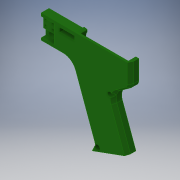
# Autodesk Inventor part: Griff_rechts
Saved by Autodesk Inventor 2019 (Build 230136000, 136)
## iProperties
Created: 2021-03-07
Part Number: Griff_rechts
Material: Generic
Document SubType Name: Modeling
Designer: Lukas
Density: 1 g/cm^3
Appearance: Default(3)
Author: Lukas
Autodesk Inventor part; units mm, degrees
ref_plane "YZ Plane" through (0, 0, 0) normal (1, 0, 0) x (0, 1, 0)
ref_plane "XZ Plane" through (0, 0, 0) normal (0, 1, 0) x (-1, 0, 0)
ref_plane "XY Plane" through (0, 0, 0) normal (0, 0, 1) x (1, 0, 0)
sketch "Sketch1" plane through (0, 0, 0) normal (0, 0, 1) x (1, 0, 0)
  line L0 (-51.5891, 42.2862) -> (-20.8072, -42.2862)
  line L1 (-20.8072, -42.2862) -> (-24.5184, -46.7089)
  line L2 (-24.5184, -46.7089) -> (-23.4923, -49.528)
  line L3 (-23.4923, -49.528) -> (23.4923, -32.427)
  line L4 (27.261, 47.2862) -> (1.261, 28.653)
  line L5 (1.261, 28.653) -> (23.4923, -32.427)
  line L6 (0, -74.8908) -> (0, 102.649) projected
  line L7 (-91.5891, 77.2862) -> (27.261, 77.2862)
  line L8 (27.261, 77.2862) -> (27.261, 47.2862)
  line L9 (-51.5891, 42.2862) -> (-91.5891, 42.2862)
  line L10 (-91.5891, 42.2862) -> (-91.5891, 77.2862)
  point P0 (0, 0)
  point P1 (-36.1981, 0)
  point P2 (0, -40.9775)
  dimension "d1" = 90
  dimension "d2" = 120
  dimension "d3" = 3
  dimension "d5" = 45
  dimension "d6" = 20
  dimension "d7" = 65
  dimension "d8" = 5
  dimension "d10" = 30
  dimension "d30" = 26
  dimension "d31" = 40
  dimension "d32" = 35
  constraints: 21 end point, 5 perpendicular, 2 midpoint, 1 horizontal, 1 horizontal alignment, 1 parallel, 1 vertical alignment
  measures "d1" distance of L0.start L0.end
  measures "d2" angle of L0 L1
  measures "d3" distance of L1.end L2.end
  measures "d5" distance between parallel lines of L5 L0
  measures "d6" angle of L6 L0
  measures "d7" distance of L4.end L3.end
  measures "d8" distance between parallel lines of L2 L0
  measures "d10" distance of L7.end L4.start
  measures "d30" distance from line of L8 L4.end
  measures "d31" distance of L0.start L9.end
  measures "d32" distance of L9.end L7.start
extrude "Extrusion1" add sketch "Sketch1" along normal blind 2.5
sketch "Sketch2" plane through (0, 0, 0) normal (0, 0, 1) x (1, 0, 0)
  line L0 (-51.5891, 42.2862) -> (-20.8072, -42.2862) projected
  line L1 (-20.8072, -42.2862) -> (-24.5184, -46.7089) projected
  line L2 (-24.5184, -46.7089) -> (-23.4923, -49.528) projected
  line L3 (-23.4923, -49.528) -> (23.4923, -32.427) projected
  line L4 (23.4923, -32.427) -> (1.261, 28.653) projected
  line L5 (1.261, 28.653) -> (27.261, 47.2862) projected
  line L6 (27.261, 47.2862) -> (27.261, 77.2862) projected
  line L7 (27.261, 77.2862) -> (-91.5891, 77.2862) projected
  circle A0 centre (-32, 28) radius 3
  circle A1 centre (-32, 28) radius 8.5
  line L8 (-91.5891, 77.2862) -> (-91.5891, 42.2862) projected
  line L9 (-91.5891, 42.2862) -> (-51.5891, 42.2862) projected
  point P0 (0, 0)
  dimension "d55" = 6
  dimension "d56" = 17
  dimension "d169" = 32
  dimension "d170" = 28
  constraints: 2 centre point, 1 coincident
  measures "d55" diameter of A0
  measures "d56" diameter of A1
  measures "d169" horizontal distance of A0.centre point (0, 0)
  measures "d170" vertical distance of point (0, 0) A0.centre
extrude "Extrusion2" add sketch "Sketch2" against normal blind 6 contours A1
sketch "Sketch3" plane through (0, 0, 0) normal (0, 0, 1) x (1, 0, 0)
  line L0 (-51.5891, 42.2862) -> (-20.8072, -42.2862) projected
  line L1 (-20.8072, -42.2862) -> (-24.5184, -46.7089) projected
  line L2 (-24.5184, -46.7089) -> (-23.4923, -49.528) projected
  line L3 (-23.4923, -49.528) -> (23.4923, -32.427) projected
  line L4 (23.4923, -32.427) -> (1.261, 28.653) projected
  line L5 (1.261, 28.653) -> (27.261, 47.2862) projected
  line L6 (27.261, 47.2862) -> (27.261, 77.2862) projected
  line L7 (27.261, 77.2862) -> (-91.5891, 77.2862) projected
  line L8 (-48.7882, 46.2862) -> (-16.4032, -42.6911)
  line L9 (-16.4032, -42.6911) -> (18.3655, -30.0363)
  line L10 (18.3655, -30.0363) -> (-3.5357, 30.1366)
  line L11 (-3.5357, 30.1366) -> (23.261, 49.3407)
  line L12 (23.261, 49.3407) -> (23.261, 77.2862)
  line L13 (27.261, 77.2862) -> (-91.5891, 77.2862) projected
  line L14 (1.261, 28.653) -> (27.261, 47.2862) projected
  line L15 (23.4923, -32.427) -> (1.261, 28.653) projected
  line L16 (-51.5891, 42.2862) -> (-20.8072, -42.2862) projected
  line L17 (-24.5184, -46.7089) -> (-20.8072, -42.2862) projected
  line L18 (-51.5891, 42.2862) -> (-20.8072, -42.2862)
  line L19 (-20.8072, -42.2862) -> (-24.5184, -46.7089)
  line L20 (-24.5184, -46.7089) -> (-23.4923, -49.528)
  line L21 (23.4923, -32.427) -> (-23.4923, -49.528)
  line L22 (-23.4923, -49.528) -> (23.4923, -32.427) projected
  line L23 (23.4923, -32.427) -> (1.261, 28.653)
  line L24 (1.261, 28.653) -> (27.261, 47.2862)
  line L25 (27.261, 77.2862) -> (27.261, 47.2862)
  line L26 (23.261, 77.2862) -> (27.261, 77.2862)
  line L27 (-91.5891, 77.2862) -> (-91.5891, 42.2862) projected
  line L28 (-91.5891, 42.2862) -> (-51.5891, 42.2862) projected
  line L29 (-91.5891, 77.2862) -> (-91.5891, 42.2862) projected
  line L30 (-51.5891, 42.2862) -> (-91.5891, 42.2862)
  line L31 (-91.5891, 42.2862) -> (-91.5891, 46.2862)
  line L32 (-91.5891, 46.2862) -> (-48.7882, 46.2862)
  point P0 (-51.5891, 77.2862)
  dimension "d20" = 4
  dimension "d21" = 4
  dimension "d22" = 4
  dimension "d23" = 4
  dimension "d24" = 4
  dimension "d33" = 4
  constraints: 32 end point, 6 perpendicular, 5 parallel, 2 point on line, 2 vertical, 1 collinear, 1 horizontal
  measures "d20" distance between parallel lines of L6 L12
  measures "d21" distance between parallel lines of L16 L8
  measures "d22" distance between parallel lines of L4 L10
  measures "d23" distance between parallel lines of L14 L11
  measures "d24" distance between parallel lines of L3 L9
  measures "d33" distance between parallel lines of L32 L28
extrude "Extrusion3" add sketch "Sketch3" against normal blind 10 contours L28 L27 L32 L8 L9 L10 L11 L12 L7 L6 L5 L4 L3 L2 L1 L0
fillet "Fillet7" radius 3 1 edges at (-40.5, 28, 0)
fillet "Fillet1" radius 6 2 edges at (7.4149, 0.0501, 0) (9.8627, 39.7386, 0)
fillet "Fillet3" radius 15 2 edges at (1.261, 28.653, -3.75) (-51.5891, 42.2862, -3.75)
fillet "Fillet2" radius 8 2 edges at (27.261, 47.2862, -3.75) (-20.8072, -42.2862, -3.75)
chamfer "Chamfer3" distance 3 angle 60 10 edges at (14.3227, -7.2338, 2.5) (4.9183, 27.5219, 2.5) (17.216, 40.0873, 2.5) (26.3772, 47.7401, 2.5) (27.261, 64.3407, 2.5) (-35.1919, -2.7647, 2.5) (-22.026, -42.0713, 2.5) (-24.1473, -46.2667, 2.5) (-53.4885, 39.5734, 2.5) (-76.8406, 42.2862, 2.5) measured on face at (-53.2017, 39.983, 2.5) measured on face at (26.761, 64.3407, 2.5) measured on face at (25.9325, 47.9685, 2.5) measured on face at (13.8529, -7.4048, 2.5) measured on face at (16.9247, 40.4937, 2.5) measured on face at (-76.8406, 42.7862, 2.5) measured on face at (4.4406, 27.6696, 2.5) measured on face at (-23.7642, -46.588, 2.5) measured on face at (-34.722, -2.5937, 2.5) measured on face at (-21.5336, -42.1581, 2.5)
sketch "Sketch4" plane through (0, 0, 0) normal (0, 0, 1) x (1, 0, 0)
  line L0 (-91.5891, 77.2862) -> (-91.5891, 46.2862) projected
  line L1 (-91.5891, 77.2862) -> (-42.0891, 77.2862)
  line L2 (-42.0891, 77.2862) -> (-42.0891, 60.2862)
  line L3 (-42.0891, 60.2862) -> (-91.5891, 60.2862)
  line L4 (-91.5891, 60.2862) -> (-91.5891, 77.2862)
  line L5 (24.261, 77.2862) -> (-91.5891, 77.2862) projected
  line L6 (-91.5891, 46.2862) -> (-48.7882, 46.2862) projected
  point P0 (0, 0)
  point P1 (11.261, 77.2862)
  point P2 (-76.5891, 52.2862)
  point P3 (-59.2913, 46.2862)
  point P4 (17.261, 77.2862)
  point P5 (27.261, 77.2862)
  dimension "d34" = 49.5
  dimension "d35" = 0
  dimension "d42" = 14
  constraints: 8 end point, 2 parallel, 1 horizontal, 1 perpendicular, 2 other
  measures "d34" distance of L1.start L1.end
  measures "d35" distance between parallel lines of L5 L1
  measures "d42" distance between parallel lines of L6 L3
extrude "Extrusion4" add sketch "Sketch4" against normal blind 10
chamfer "Chamfer1" distance 1 distance2 4 1 edges at (-42.0891, 77.2862, -5) measured on face at (-42.0891, 76.7862, -5)
chamfer "Chamfer4" distance 10 angle 45 1 edges at (-16.4032, -42.6911, -5)
sketch "Sketch5" plane through (-91.5891, 77.2862, 0) normal (-1, 0, 0) x (0, 0, 1)
  circle A0 centre (-13, -7.5) radius 5
  line L0 (-10, -17) -> (-10, 0) projected
  line L1 (2.5, 0) -> (-10, 0) projected
  point P0 (0, -77.2862)
  dimension "d39" = 10
  dimension "d147" = 7.5
  dimension "d148" = 3
  constraints: 1 centre point
  measures "d39" diameter of A0
  measures "d147" distance from line of L1 A0.centre
  measures "d148" distance from line of L0 A0.centre
extrude "Extrusion5" cut sketch "Sketch5" against normal up to surface (49.5 mm away)
sketch "Sketch20" plane through (0, 0, -10) normal (0, 0, -1) x (-1, 0, 0)
  line L0 (42.0891, 73.7862) -> (91.5891, 73.7862) projected
  line L1 (42.0891, 65.7862) -> (42.0891, 73.7862) projected
  line L2 (91.5891, 65.7862) -> (42.0891, 65.7862) projected
  line L3 (91.5891, 73.7862) -> (91.5891, 65.7862) projected
  line L4 (42.0891, 73.7862) -> (91.5891, 73.7862) projected
  line L5 (91.5891, 73.7862) -> (91.5891, 77.2862) projected
  line L6 (91.5891, 77.2862) -> (46.0891, 77.2862) projected
  line L7 (42.0891, 76.2862) -> (46.0891, 77.2862) projected
  line L8 (42.0891, 76.2862) -> (42.0891, 73.7862) projected
  line L9 (91.5891, 65.7862) -> (42.0891, 65.7862) projected
  line L10 (42.0891, 65.7862) -> (42.0891, 60.2862) projected
  line L11 (42.0891, 60.2862) -> (91.5891, 60.2862) projected
  line L12 (91.5891, 60.2862) -> (91.5891, 65.7862) projected
  line L13 (47.0891, 72.7862) -> (67.0891, 72.7862)
  line L14 (67.0891, 72.7862) -> (67.0891, 66.7862)
  line L15 (67.0891, 66.7862) -> (47.0891, 66.7862)
  line L16 (47.0891, 66.7862) -> (47.0891, 72.7862)
  point P0 (0, 0)
  point P1 (47.0891, 69.7862)
  point P2 (42.0891, 69.7862)
  dimension "d135" = 5
  dimension "d136" = 6
  dimension "d137" = 20
  constraints: 8 end point, 2 midpoint, 2 parallel, 1 horizontal, 1 horizontal alignment, 1 perpendicular
  measures "d135" distance between parallel lines of L1 L16
  measures "d136" distance of L15.end L13.start
  measures "d137" distance of L13.start L13.end
extrude "Extrusion21" cut sketch "Sketch20" against normal through all contours L13 L14 L15 L16
sketch "Sketch21" plane through (0, 0, 0) normal (0, 0, -1) x (-1, 0, 0)
  line L0 (48.7882, 46.2862) -> (91.5891, 46.2862) projected
  line L1 (91.5891, 60.2862) -> (71.5891, 60.2862)
  line L2 (71.5891, 60.2862) -> (71.5891, 46.2862)
  line L3 (71.5891, 46.2862) -> (91.5891, 46.2862)
  line L4 (91.5891, 46.2862) -> (91.5891, 60.2862)
  point P0 (0, 0)
  point P1 (42.3941, 46.2862)
  point P2 (42.4032, 46.2862)
  dimension "d140" = 20
  constraints: 8 end point, 2 parallel, 1 horizontal, 1 perpendicular, 1 point on line
  measures "d140" distance between parallel lines of L4 L2
extrude "Extrusion22" add sketch "Sketch21" along normal up to surface (10 mm away)
sketch "Sketch23" plane through (-91.5891, 45.2862, 2.5) normal (-1, 0, 0) x (0, 0, 1)
  line L0 (-5.1962, -3) -> (-12.5, -3) projected
  line L1 (-12.5, -3) -> (-12.5, 20.5) projected
  line L2 (-11.5, -3) -> (-12.5, -3)
  line L3 (-12.5, -3) -> (-12.5, 0)
  line L4 (-12.5, 0) -> (-11.5, 0)
  line L5 (-11.5, 0) -> (-11.5, -3)
  arc A0 (-12.5, 20.5) -> (-12.5, 28.5) centre (-15.5, 24.5) ccw projected
  line L6 (-12.5, -3) -> (-12.5, 20.5) projected
  line L7 (-5.1962, -3) -> (-12.5, -3) projected
  line L8 (0, 0) -> (-5.1962, -3) projected
  line L9 (0, 32) -> (0, 0) projected
  line L10 (0, 32) -> (-12.5, 32) projected
  line L11 (-12.5, 28.5) -> (-12.5, 32) projected
  line L12 (0, 32) -> (0, 0) projected
  line L13 (0, 3) -> (-6, 3)
  line L14 (-6, 3) -> (-6, 13)
  line L15 (-6, 13) -> (0, 13)
  line L16 (0, 13) -> (0, 3)
  line L17 (0, 13) -> (-3, 13)
  line L18 (-3, 13) -> (-3, 28)
  line L19 (-3, 28) -> (0, 28)
  line L20 (0, 28) -> (0, 13)
  point P0 (-2.5, -45.2862)
  dimension "d149" = 3
  dimension "d150" = 1
  dimension "d151" = 6
  dimension "d152" = 10
  dimension "d153" = 15
  dimension "d154" = 3
  dimension "d155" = 3
  constraints: 24 end point, 6 parallel, 3 horizontal, 3 perpendicular, 3 point on line
  measures "d149" distance of L4.end L2.start
  measures "d150" distance of L3.end L4.end
  measures "d151" distance between parallel lines of L13 L0
  measures "d152" distance of L13.end L14.end
  measures "d153" distance of L17.end L18.end
  measures "d154" distance of L18.end L19.end
  measures "d155" distance between parallel lines of L14 L18
extrude "Extrusion24" cut sketch "Sketch23" against normal blind 17.25 contours L0 L1 L4 L5 | L13 L14 L15 L9 | L15 L18 L19 L9
sketch "Sketch24" plane through (-91.5891, 58.2862, -0.5) normal (0, 0, 1) x (1, 0, 0)
  circle A0 centre (13, 11) radius 1.35
  circle A1 centre (13, 4) radius 1.35
  circle A2 centre (3, 4) radius 1.35
  circle A3 centre (3, 11) radius 1.35
  line L0 (0, 0) -> (0, 15) projected
  line L1 (0, 0) -> (17.25, 0) projected
  line L2 (0, 15) -> (17.25, 15) projected
  point P0 (91.5891, -58.2862)
  dimension "d158" = 3
  dimension "d159" = 10
  dimension "d160" = 4
  dimension "d161" = 4
  dimension "d162" = 2.7
  constraints: 4 centre point, 3 equal radius, 2 horizontal alignment, 2 vertical alignment
  measures "d158" distance from line of L0 A3.centre
  measures "d159" distance of A0.centre A3.centre
  measures "d160" distance from line of L1 A2.centre
  measures "d161" distance from line of L2 A0.centre
  measures "d162" diameter of A3
extrude "Extrusion25" cut sketch "Sketch24" against normal blind 9
sketch "Sketch25" plane through (23.261, 77.2862, -10) normal (0, 1, 0) x (1, 0, 0)
  line L0 (-114.8501, 0) -> (-69.3501, 0) projected
  line L1 (-114.8501, 0) -> (-69.3501, 0)
  line L2 (-69.3501, 0) -> (-69.3501, -2)
  line L3 (-69.3501, -2) -> (-114.8501, -2)
  line L4 (-114.8501, -2) -> (-114.8501, 0)
  point P0 (-23.261, -10)
  dimension "d165" = 45.5
  dimension "d166" = 2
  constraints: 8 end point, 2 parallel, 1 horizontal, 1 perpendicular
  measures "d165" distance of L2.end L3.end
  measures "d166" distance of L1.end L2.end
extrude "Extrusion26" cut sketch "Sketch25" against normal blind 7.5
sketch "Sketch26" plane through (0, 0, -10) normal (0, 0, -1) x (-1, 0, 0)
  circle A0 centre (-1, 28) radius 1.6
  circle A1 centre (16, -42) radius 1.6
  circle A2 centre (83.5891, 52.2862) radius 1.6
  line L0 (62.0922, 42.2862) -> (74.3391, 42.2862) projected
  line L1 (91.5891, 45.2862) -> (91.5891, 65.7862) projected
  point P0 (0, 0)
  dimension "d174" = 1
  dimension "d175" = 28
  dimension "d176" = 3.2
  dimension "d182" = 42
  dimension "d183" = 16
  dimension "d187" = 10
  dimension "d188" = 8
  constraints: 3 centre point, 2 equal radius
  measures "d174" horizontal distance of point (0, 0) A0.centre
  measures "d175" vertical distance of point (0, 0) A0.centre
  measures "d176" diameter of A0
  measures "d182" vertical distance of A1.centre point (0, 0)
  measures "d183" horizontal distance of A1.centre point (0, 0)
  measures "d187" distance from line of L0 A2.centre
  measures "d188" distance from line of L1 A2.centre
extrude "Extrusion27" cut sketch "Sketch26" against normal through all
sketch "Sketch27" plane through (0, 0, 2.5) normal (0, 0, 1) x (1, 0, 0)
  arc A0 (2.2473, 29.0021) -> (1.576, 26.5073) centre (1, 28) ccw projected
  circle A1 centre (1, 28) radius 1.6 projected
  circle A2 centre (1, 28) radius 3.5
  circle A3 centre (-16, -42) radius 1.6 projected
  circle A4 centre (-16, -42) radius 1.6 projected
  circle A5 centre (-16, -42) radius 1.6 projected
  circle A6 centre (-16, -42) radius 3.5
  point P0 (0, 0)
  dimension "d179" = 7
  constraints: 2 centre point, 2 coincident, 1 equal radius, 1 other
  measures "d179" diameter of A2
extrude "Extrusion28" cut sketch "Sketch27" against normal blind 5
chamfer "Chamfer5" distance 2.5 angle 45 1 edges at (-81.9891, 52.2862, -3.5)
equation "\"d21\" = d20"
equation "\"d22\" = d20"
equation "\"d23\" = d20"
equation "\"d24\" = d20"
equation "\"d33\" = d20"
body "Solid1"
